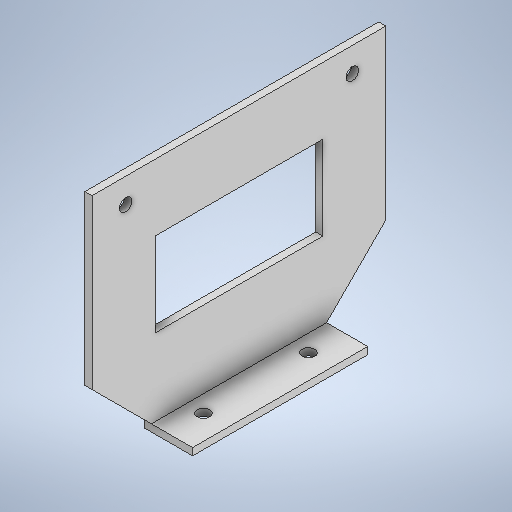
# Autodesk Inventor part: servo mount
Saved by Autodesk Inventor 2025.2 (Build 292293000, 293)
## iProperties
Created: 2025-05-22
Part Number: servo mount
Material: Generic
Document SubType Name: Modeling
Designer: Verchasv
Density: 1 g/cm^3
Appearance: Default
Author: Verchasv
Autodesk Inventor part; units mm, degrees
ref_plane "YZ Plane" through (0, 0, 0) normal (1, 0, 0) x (0, 1, 0)
ref_plane "XZ Plane" through (0, 0, 0) normal (0, 1, 0) x (-1, 0, 0)
ref_plane "XY Plane" through (0, 0, 0) normal (0, 0, 1) x (1, 0, 0)
sketch "Sketch1" plane through (0, 0, 0) normal (0, 1, 0) x (-1, 0, 0)
  line L0 (0, 12.5) -> (0, -12.5) construction
  line L1 (-1.5, 12.5) -> (-1.5, -12.5)
  line L2 (1.5, -12.5) -> (1.5, 12.5)
  arc A0 (1.5, 12.5) -> (-1.5, 12.5) centre (0, 12.5) ccw
  arc A1 (-1.5, -12.5) -> (1.5, -12.5) centre (0, -12.5) ccw
  circle A2 centre (0, -12.5) radius 1.5
  circle A3 centre (0, 12.5) radius 1.5
  line L3 (-5.7579, 20.8654) -> (5.7579, 20.8654)
  line L4 (5.7579, 20.8654) -> (5.7579, -20.8654)
  line L5 (5.7579, -20.8654) -> (-5.7579, -20.8654)
  line L6 (-5.7579, -20.8654) -> (-5.7579, 20.8654)
  line L7 (-5.7579, 20.8654) -> (5.7579, -20.8654) construction
  line L8 (5.7579, 20.8654) -> (-5.7579, -20.8654) construction
  point P0 (0, 0)
  dimension "d0" = 12.5
  dimension "d1" = 3
  dimension "d2" = 3
  dimension "d3" = 3
  constraints: 20 end point, 4 centre point, 4 point on circle, 4 tangent, 3 midpoint, 3 parallel, 2 coincident, 1 horizontal, 1 perpendicular, 1 vertical
  measures "d0" distance of point (0, 0) L0.end
  measures "d1" diameter of A1
  measures "d2" diameter of A2
  measures "d3" diameter of A3
extrude "Extrusion1" add sketch "Sketch1" along normal blind 1.7 contours A3 L2 A2 L1 | L3 L4 L5 L6
sketch "Sketch2" plane through (-5.7579, 0, -20.8654) normal (-1, 0, 0) x (0, 0, 1)
  line L0 (40.8654, 20) -> (0.8654, 20)
  line L1 (0.8654, 20) -> (0.8654, 40)
  line L2 (0.8654, 40) -> (40.8654, 40)
  line L3 (40.8654, 40) -> (40.8654, 20)
  line L4 (40.8654, 20) -> (0.8654, 40) construction
  line L5 (0.8654, 20) -> (40.8654, 40) construction
  line L6 (41.7309, 0) -> (0, 0) projected
  circle A0 centre (47.8654, 50) radius 1.5
  circle A1 centre (-6.1346, 50) radius 1.5
  line L7 (0, 1.7) -> (41.7309, 1.7) projected
  line L8 (41.7309, 1.7) -> (55.873, 15.8421)
  line L9 (41.7309, 1.7) -> (61.7309, 1.7) construction
  line L10 (55.873, 15.8421) -> (55.873, 55.8421)
  line L11 (55.873, 15.8421) -> (95.873, 15.8421) construction
  line L12 (0, 1.7) -> (-14.1421, 15.8421)
  line L13 (0, 1.7) -> (20, 1.7) construction
  line L14 (-14.1421, 15.8421) -> (-14.1421, 55.8421)
  line L15 (-14.1421, 55.8421) -> (55.873, 55.8421)
  point P0 (20.8654, 0)
  point P1 (20.8654, 30)
  dimension "d6" = 40
  dimension "d7" = 20
  dimension "d8" = 30
  dimension "d9" = 3
  dimension "d10" = 3
  dimension "d11" = 50
  dimension "d12" = 50
  dimension "d13" = 54
  dimension "d14" = 27
  dimension "d15" = 20
  dimension "d16" = 45
  dimension "d17" = 40
  dimension "d18" = 90
  dimension "d19" = 20
  dimension "d20" = 135
  dimension "d21" = 40
  constraints: 28 end point, 4 horizontal, 3 equal length, 2 centre point, 2 midpoint, 2 parallel, 2 vertical, 1 perpendicular
  measures "d6" distance of L1.end L2.end
  measures "d7" distance of L0.end L1.end
  measures "d8" distance from line of L6 point (20.865, 30)
  measures "d9" diameter of A0
  measures "d10" diameter of A1
  measures "d11" distance from line of L6 A1.centre
  measures "d12" distance from line of L6 A0.centre
  measures "d13" distance of A1.centre A0.centre
  measures "d14" horizontal distance of point (20.865, 30) A0.centre
  measures "d15" distance of L7.end L8.end
  measures "d16" angle of L9 L8
  measures "d17" distance of L8.end L10.end
  measures "d18" angle of L11 L10
  measures "d19" distance of L7.start L12.end
  measures "d20" angle of L13 L12
  measures "d21" distance of L12.end L14.end
extrude "Extrusion2" add sketch "Sketch2" against normal blind 1.7
body "Solid1"
